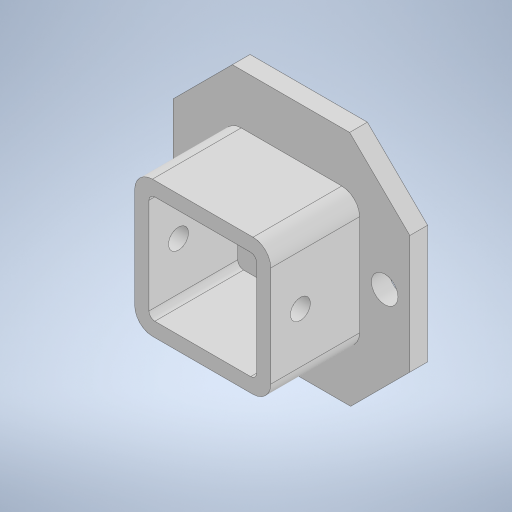
# Autodesk Inventor part: rod_fixture_vp13
Saved by Autodesk Inventor 2024 (Build 280153000, 153)
## iProperties
Created: 2024-10-07
Part Number: rod_fixture_vp13
Material: 一般
Document SubType Name: Modeling
Designer: 1412z
Density: 1 g/cm^3
Appearance: 既定
Author: 1412z
Autodesk Inventor part; units mm, degrees
ref_plane "YZ Plane" through (0, 0, 0) normal (1, 0, 0) x (0, 1, 0)
ref_plane "XZ Plane" through (0, 0, 0) normal (0, 1, 0) x (-1, 0, 0)
ref_plane "XY Plane" through (0, 0, 0) normal (0, 0, 1) x (1, 0, 0)
sketch "スケッチ1" plane through (0, 0, 0) normal (0, 0, 1) x (1, 0, 0)
  line L0 (-9.1, 9.1) -> (9.1, 9.1)
  line L1 (9.1, 9.1) -> (9.1, -9.1)
  line L2 (9.1, -9.1) -> (-9.1, -9.1)
  line L3 (-9.1, -9.1) -> (-9.1, 9.1)
  line L4 (-9.1, 9.1) -> (9.1, -9.1) construction
  line L5 (9.1, 9.1) -> (-9.1, -9.1) construction
  line L6 (-11.5, 11.5) -> (11.5, 11.5)
  line L7 (11.5, 11.5) -> (11.5, -11.5)
  line L8 (11.5, -11.5) -> (-11.5, -11.5)
  line L9 (-11.5, -11.5) -> (-11.5, 11.5)
  line L10 (-11.5, 11.5) -> (11.5, -11.5) construction
  line L11 (11.5, 11.5) -> (-11.5, -11.5) construction
  point P0 (0, 0)
  dimension "d0" = 18.2
  dimension "d1" = 18.2
  dimension "d2" = 23
  dimension "d3" = 23
  constraints: 24 end point, 4 midpoint, 4 parallel, 2 horizontal, 2 perpendicular
  measures "d0" distance of L1.end L2.end
  measures "d1" distance of L0.end L1.end
  measures "d2" distance of L7.end L8.end
  measures "d3" distance of L6.end L7.end
extrude "押し出し1" add sketch "スケッチ1" along normal blind 15
sketch "スケッチ2" plane through (-11.5, -11.5, 0) normal (-1, 0, 0) x (0, 0, 1)
  circle A0 centre (10, 11.5) radius 1.7
  point P0 (0, 11.5)
  dimension "d6" = 3.4
  constraints: 1 centre point
  measures "d6" diameter of A0
extrude "押し出し2" cut sketch "スケッチ2" against normal blind 30
sketch "スケッチ3" plane through (0, 0, 0) normal (0, 0, -1) x (-1, 0, 0)
  line L0 (20, 20) -> (-20, 20)
  line L1 (-20, 20) -> (-20, -20)
  line L2 (-20, -20) -> (20, -20)
  line L3 (20, -20) -> (20, 20)
  line L4 (20, 20) -> (-20, -20) construction
  line L5 (-20, 20) -> (20, -20) construction
  point P0 (0, 0)
  dimension "d9" = 40
  dimension "d10" = 40
  constraints: 12 end point, 2 midpoint, 2 parallel, 1 horizontal, 1 perpendicular
  measures "d9" distance of L2.end L1.end
  measures "d10" distance of L1.end L0.end
extrude "押し出し3" add sketch "スケッチ3" along normal blind 3
sketch "スケッチ4" plane through (0, 0, 0) normal (0, 0, 1) x (1, 0, 0)
  point P0 (0, 0)
sketch "スケッチ5" plane through (0, 0, 0) normal (0, 0, 1) x (1, 0, 0)
  circle A0 centre (-15.75, 0) radius 2.25
  circle A1 centre (15.75, 0) radius 2.25
  point P0 (0, 0)
  dimension "d13" = 4.5
  dimension "d14" = 4.5
  constraints: 2 centre point
  measures "d13" diameter of A0
  measures "d14" diameter of A1
extrude "押し出し4" cut sketch "スケッチ5" against normal blind 3
sketch "スケッチ6" plane through (0, 0, 0) normal (0, 0, 1) x (1, 0, 0)
  line L0 (-20, -20) -> (-20, 20) projected
  line L1 (-20, 20) -> (20, 20) projected
  line L2 (-20, 10) -> (-20, 20)
  line L3 (-20, 20) -> (-10, 20)
  line L4 (-10, 20) -> (-20, 10)
  line L5 (19.8208, 20) -> (9.8208, 20)
  line L6 (20, 20) -> (20, -20) projected
  line L7 (20, 20) -> (20, 10)
  line L8 (20, 10) -> (9.8208, 20)
  line L9 (-20, -20) -> (-20, -10)
  line L10 (-20, -20) -> (-10, -20)
  line L11 (20, -20) -> (-20, -20) projected
  line L12 (-10, -20) -> (-20, -10)
  line L13 (20, -20) -> (10, -20)
  line L14 (20, -20) -> (20, -10)
  line L15 (10, -20) -> (20, -10)
  point P0 (0, 0)
  dimension "d17" = 10
  dimension "d18" = 10
  dimension "d19" = 10
  dimension "d20" = 10
  dimension "d21" = 10
  dimension "d22" = 10
  constraints: 24 end point, 8 point on line, 2 perpendicular
  measures "d17" distance of L0.end L3.end
  measures "d18" distance of L5.start L5.end
  measures "d19" distance of L1.end L7.end
  measures "d20" distance of L0.start L9.end
  measures "d21" distance of L0.start L10.end
  measures "d22" distance of L6.end L13.end
extrude "押し出し5" cut sketch "スケッチ6" against normal blind 3 contours L0 L12 L10 | L0 L1 L4 | L15 L6 L11 | L1 L6 L8
fillet "フィレット1" radius 3 4 edges at (-11.5, 11.5, 7.5) (11.5, 11.5, 7.5) (11.5, -11.5, 7.5) (-11.5, -11.5, 7.5)
fillet "フィレット2" radius 1 4 edges at (-9.1, 9.1, 7.5) (9.1, 9.1, 7.5) (-9.1, -9.1, 7.5) (9.1, -9.1, 7.5)
